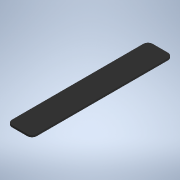
# Autodesk Inventor part: antenna
Saved by Autodesk Inventor 2022 (Build 260153000, 153)
## iProperties
Created: 2025-01-04
Part Number: antenna
Material: Типовые
Document SubType Name: Modeling
Designer: akap
Density: 1 g/cm^3
Appearance: По умолчанию
Author: akap
Autodesk Inventor part; units mm, degrees
ref_plane "YZ Plane" through (0, 0, 0) normal (1, 0, 0) x (0, 1, 0)
ref_plane "XZ Plane" through (0, 0, 0) normal (0, 1, 0) x (-1, 0, 0)
ref_plane "XY Plane" through (0, 0, 0) normal (0, 0, 1) x (1, 0, 0)
sketch "Эскиз1" plane through (0, 0, 0) normal (0, 1, 0) x (-1, 0, 0)
  line L0 (4.5, 25.5) -> (-4.5, 25.5)
  line L1 (-4.5, 25.5) -> (-4.5, -25.5)
  line L2 (-4.5, -25.5) -> (4.5, -25.5)
  line L3 (4.5, -25.5) -> (4.5, 25.5)
  line L4 (4.5, 25.5) -> (-4.5, -25.5) construction
  line L5 (-4.5, 25.5) -> (4.5, -25.5) construction
  point P0 (0, 0)
  dimension "d0" = 9
  dimension "d1" = 51
  constraints: 12 end point, 2 midpoint, 2 parallel, 1 horizontal, 1 perpendicular
  measures "d0" distance of L2.end L1.end
  measures "d1" distance of L1.end L0.end
extrude "Выдавливание1" add sketch "Эскиз1" along normal blind 0.66
fillet "Сопряжение1" radius 1.7 4 edges at (4.5, 0.33, 25.5) (-4.5, 0.33, 25.5) (-4.5, 0.33, -25.5) (4.5, 0.33, -25.5)
